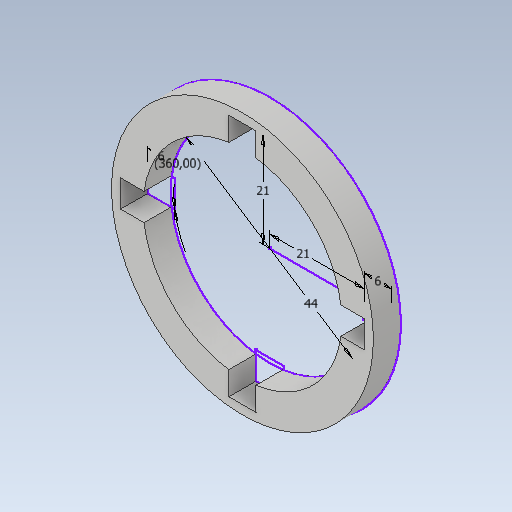
# Autodesk Inventor part: Part2
Saved by Autodesk Inventor 2020 (Build 240168000, 168)
## iProperties
Created: 2020-12-21
Part Number: Part2
Material: Generic
Document SubType Name: Modeling
Designer: Dell
Density: 1 g/cm^3
Appearance: Default
Author: Dell
Autodesk Inventor part; units mm, degrees
ref_plane "YZ Plane" through (0, 0, 0) normal (1, 0, 0) x (0, 1, 0)
ref_plane "XZ Plane" through (0, 0, 0) normal (0, 1, 0) x (-1, 0, 0)
ref_plane "XY Plane" through (0, 0, 0) normal (0, 0, 1) x (1, 0, 0)
sketch "Sketch1" plane through (0, 0, 0) normal (0, 0, 1) x (1, 0, 0)
  line L0 (-25, -3) -> (-25, 3)
  line L1 (17, -3) -> (17, 3)
  line L2 (-25, -3) -> (-31, -3)
  line L3 (-31, -3) -> (-31, 3)
  line L4 (-31, 3) -> (-25, 3)
  line L5 (-25, 3) -> (-25, -3)
  line L6 (17, -3) -> (23, -3)
  line L7 (23, -3) -> (23, 3)
  line L8 (23, 3) -> (17, 3)
  line L9 (17, 3) -> (17, -3)
  circle A0 centre (-4, 0) radius 29
  line L10 (-1, -21) -> (-1, -27)
  line L11 (-1, -27) -> (-7, -27)
  line L12 (-7, -27) -> (-7, -21)
  line L13 (-7, -21) -> (-1, -21)
  line L14 (17, 3) -> (23, 3)
  line L15 (23, 3) -> (23, -3)
  line L16 (23, -3) -> (17, -3)
  line L17 (17, -3) -> (17, 3)
  line L18 (-7, 21) -> (-7, 27)
  line L19 (-7, 27) -> (-1, 27)
  line L20 (-1, 27) -> (-1, 21)
  line L21 (-1, 21) -> (-7, 21)
  circle A1 centre (-4, 0) radius 22
  line L22 (-4, 0) -> (17, 0)
  point P0 (-7, -21)
  point P1 (-1, 21)
  dimension "d10" = 6
  dimension "d12" = 6
  dimension "d21" = 360
  dimension "d25" = 44
  dimension "d29" = 21
  dimension "d30" = 21
  constraints: 46 end point, 4 parallel, 2 centre point, 2 horizontal, 2 perpendicular, 1 coincident, 1 midpoint, 37 other
  measures "d10" distance of L3.end L4.end
  measures "d12" distance of L8.end L7.end
  measures "d25" diameter of A1
  measures "d29" distance of L22.start L22.end
  measures "d30" distance from line of A0.centre L21
extrude "Extrusion1" add sketch "Sketch1" along normal blind 6
body "Solid1"
